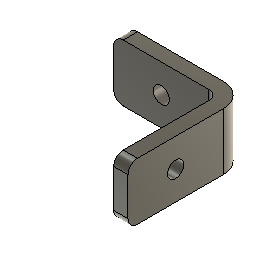
メインロボット ver2 v8 (Autodesk Fusion 360 archive; units mm, degrees)
design "L字固定具"
Autodesk Fusion 360 part; units mm, degrees
sketch "スケッチ1" plane through (0, 0, 0) normal (0, 0, 1) x (1, 0, 0)
  line L0 (0, 0) -> (5, 0)
  line L1 (5, 0) -> (5, 22)
  line L2 (5, 22) -> (0, 22)
  line L3 (0, 22) -> (0, 0)
  line L4 (5, 22) -> (-20, 22)
  line L5 (-20, 22) -> (-20, 25)
  line L6 (-20, 25) -> (5, 25)
  line L7 (5, 25) -> (5, 22)
  constraint horizontal L0
  constraint vertical L1
  constraint horizontal L2
  constraint vertical L3
  constraint coincident L0.start L3.end
  constraint horizontal L4
  constraint vertical L5
  constraint horizontal L6
  constraint vertical L7
extrude "押し出し1" add sketch "スケッチ1" along normal blind 12
sketch "スケッチ2" plane through (5, 0, 0) normal (1, 0, 0) x (0, 1, 0)
  line L0 (0, 0) -> (25, 0)
  line L1 (25, 0) -> (25, 12)
  line L2 (25, 12) -> (0, 12)
  line L3 (0, 12) -> (0, 0)
  line L4 (20, 0) -> (0, 0)
  line L5 (0, 0) -> (0, 12)
  line L6 (0, 12) -> (20, 12)
  line L7 (20, 12) -> (20, 0)
  line L8 (20, 6) -> (0, 6) construction
  line L9 (10, 12) -> (10, 0) construction
  circle A0 centre (10, 6) radius 1.7
  dimension "d3" = 3.4
  constraint horizontal L4
  constraint vertical L5
  constraint horizontal L6
  constraint vertical L7
  constraint coincident L2.end L3.start
  constraint coincident L0 L4.start
  constraint midpoint L7 L8.start
  constraint midpoint L5 L8.end
  constraint midpoint L6 L9.start
  constraint midpoint L4 L9.end
  constraint midpoint L8 A0.centre
  measures "d3" diameter of A0
extrude "押し出し2" cut sketch "スケッチ2" against normal blind 5 contours A0
sketch "スケッチ3" plane through (0, 25, 0) normal (0, 1, 0) x (-1, 0, 0)
  line L0 (-5, 0) -> (20, 0)
  line L1 (20, 0) -> (20, 12)
  line L2 (20, 12) -> (-5, 12)
  line L3 (-5, 12) -> (-5, 0)
  line L4 (0, 0) -> (20, 0)
  line L5 (20, 0) -> (20, 12)
  line L6 (20, 12) -> (0, 12)
  line L7 (0, 12) -> (0, 0)
  line L8 (0, 6) -> (20, 6) construction
  line L9 (10, 12) -> (10, 0) construction
  circle A0 centre (10, 6) radius 1.7
  dimension "d6" = 3.4
  constraint horizontal L4
  constraint vertical L5
  constraint horizontal L6
  constraint vertical L7
  constraint coincident L1.end L2.start
  constraint coincident L4.start L7.end
  constraint midpoint L7 L8.start
  constraint midpoint L5 L8.end
  constraint midpoint L6 L9.start
  constraint midpoint L4 L9.end
  constraint midpoint L9 A0.centre
  measures "d6" diameter of A0
extrude "押し出し3" cut sketch "スケッチ3" against normal blind 5 contours A0
fillet "フィレット1" radius 5 1 edges at (5, 25, 6)
fillet "フィレット1" radius 2 1 edges at (0, 22, 6)
fillet "フィレット1" radius 2 4 edges at (-20, 23.5, 12) (-20, 23.5, 0) (2.5, 0, 12) (2.5, 0, 0)
move_face "面をオフセット1" offset -2 1 faces at (0, 17.2333, 6)

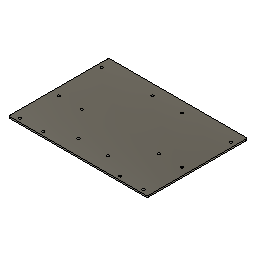
design "下板"
Autodesk Fusion 360 part; units mm, degrees
sketch "スケッチ1" plane through (0, 0, 0) normal (0, 0, 1) x (1, 0, 0)
  line L0 (0, 0) -> (180, 0)
  line L1 (180, 0) -> (180, -100)
  line L2 (180, -100) -> (0, -100)
  line L3 (0, -100) -> (0, 0)
  line L4 (0, -50) -> (180, -50) construction
  line L5 (10, -50) -> (10, -25) construction
  line L6 (10, -25) -> (40, -25) construction
  line L7 (40, -25) -> (40, -50) construction
  line L8 (90, 0) -> (90, -100) construction
  line L9 (10, -50) -> (10, -75) construction
  line L10 (10, -75) -> (40, -75) construction
  line L11 (40, -75) -> (40, -50) construction
  line L12 (140, -75) -> (140, -50) construction
  line L13 (140, -25) -> (140, -50) construction
  line L14 (170, -25) -> (140, -25) construction
  line L15 (170, -50) -> (170, -25) construction
  line L16 (170, -50) -> (170, -75) construction
  line L17 (170, -75) -> (140, -75) construction
  circle A0 centre (10, -25) radius 1.6
  circle A1 centre (40, -25) radius 1.6
  circle A2 centre (10, -75) radius 1.6
  circle A3 centre (40, -75) radius 1.6
  circle A4 centre (170, -25) radius 1.6
  circle A5 centre (140, -25) radius 1.6
  circle A6 centre (140, -75) radius 1.6
  circle A7 centre (170, -75) radius 1.6
  line L18 (40, -37.5) -> (35, -37.5)
  line L19 (35, -37.5) -> (35, -65)
  line L20 (35, -65) -> (45, -65)
  line L21 (45, -65) -> (45, -37.5)
  line L22 (45, -37.5) -> (40, -37.5)
  line L23 (145, -65) -> (135, -65)
  line L24 (135, -65) -> (135, -37.5)
  line L25 (135, -37.5) -> (140, -37.5)
  line L26 (140, -37.5) -> (145, -37.5)
  line L27 (145, -37.5) -> (145, -65)
  line L28 (90, 0) -> (64.5, 0) construction
  line L29 (64.5, 0) -> (64.5, -100) construction
  line L30 (115.5, 0) -> (115.5, -100) construction
  line L31 (64.5, -50) -> (64.5, -9) construction
  line L32 (115.5, -91) -> (115.5, -79)
  circle A8 centre (5, -5) radius 1.6
  circle A9 centre (175, -5) radius 1.6
  circle A10 centre (5, -95) radius 1.6
  circle A11 centre (175, -95) radius 1.6
  line L33 (0, -10) -> (180, -10)
  line L34 (180, -90) -> (0, -90)
  line L35 (0, -80) -> (180, -80)
  line L36 (0, -20) -> (180, -20)
  line L37 (0, 0) -> (180, 0)
  line L38 (180, 0) -> (180, 50)
  line L39 (180, 50) -> (0, 50)
  line L40 (0, 50) -> (0, 0)
  line L41 (90, -60) -> (109.25, -60)
  line L42 (109.25, -60) -> (70.75, -60)
  line L43 (70.75, -60) -> (70.75, 36)
  line L44 (70.75, 36) -> (109.25, 36)
  line L45 (109.25, 36) -> (109.25, -60)
  line L46 (90, -60) -> (90, -80)
  circle A12 centre (70.75, -60) radius 1.6
  circle A13 centre (109.25, -60) radius 1.6
  circle A14 centre (70.75, 36) radius 1.6
  circle A15 centre (109.25, 36) radius 1.6
  line L47 (0, 50) -> (0, 35)
  line L48 (0, 35) -> (180, 35)
  line L49 (0, 35) -> (6, 35)
  circle A16 centre (6, 35) radius 1.6
  circle A17 centre (174, 35) radius 1.6
  dimension "d1" = 180
  dimension "d2" = 100
  dimension "d3" = 3.2
  dimension "d4" = 3.2
  dimension "d7" = 5
  dimension "d8" = 5
  dimension "d9" = 25.5
  dimension "d10" = 41
  dimension "d17" = 3.2
  dimension "d22" = 19.25
  dimension "d23" = 38.5
  dimension "d24" = 96
  dimension "d25" = 20
  dimension "d26" = 3.2
  dimension "d27" = 3.2
  dimension "d28" = 3.2
  dimension "d29" = 3.2
  dimension "d30" = 15
  dimension "d31" = 3.2
  constraint horizontal L0
  constraint vertical L1
  constraint horizontal L2
  constraint vertical L3
  constraint coincident L0.start L3.end
  constraint midpoint L3 L4.start
  constraint midpoint L1 L4.end
  constraint coincident L4 L5.start
  constraint perpendicular L4 L5
  constraint perpendicular L3 L6
  constraint coincident L4 L7.end
  constraint perpendicular L4 L7
  constraint midpoint L0 L8.start
  constraint midpoint L2 L8.end
  constraint symmetric L4 L5.start L9.start
  constraint symmetric L4 L5.end L9.end
  constraint symmetric L4 L6.end L10.end
  constraint symmetric L4 L7.end L11.end
  constraint symmetric L5.start L8 L15.start
  constraint symmetric L5.end L8 L14.start
  constraint symmetric L6.end L8 L13.start
  constraint symmetric L7.end L8 L12.end
  constraint symmetric L8 L5.start L15.start
  constraint symmetric L8 L9.end L16.end
  constraint symmetric L8 L10.end L12.start
  constraint symmetric L8 L7.end L12.end
  constraint coincident L5.end L6.start
  constraint coincident L6.end L7.start
  constraint symmetric L4 A0 A2
  constraint symmetric L4 A1 A3
  constraint symmetric L8 A0 A4
  constraint symmetric L8 A1 A5
  constraint symmetric L8 A2 A7
  constraint symmetric L8 A3 A6
  constraint midpoint L7 L18.start
  constraint perpendicular L7 L18
  constraint perpendicular L4 L19
  constraint perpendicular L11 L20
  constraint perpendicular L20 L21
  constraint perpendicular L7 L22
  constraint symmetric L8 L18.start L25.end
  constraint symmetric L8 L18.end L26.end
  constraint symmetric L8 L19.end L23.start
  constraint symmetric L8 L20.end L23.end
  constraint symmetric L8 L21.end L24.end
  constraint perpendicular L8 L28
  constraint coincident L2 L29.end
  constraint perpendicular L2 L29
  constraint symmetric L8 L28.end L30.start
  constraint symmetric L8 L29.end L30.end
  constraint midpoint L29 L31.start
  constraint perpendicular L4 L31
  constraint symmetric L8 A8 A9
  constraint symmetric L4 A8 A10
  constraint symmetric L4 A9 A11
  constraint coincident L3 L33.start
  constraint coincident L1 L33.end
  constraint perpendicular L1 L33
  constraint coincident L1 L34.start
  constraint coincident L3 L34.end
  constraint perpendicular L3 L34
  constraint coincident L3 L35.start
  constraint coincident L1 L35.end
  constraint perpendicular L1 L35
  constraint coincident L3 L36.start
  constraint coincident L1 L36.end
  constraint perpendicular L1 L36
  constraint horizontal L37
  constraint vertical L38
  constraint horizontal L39
  constraint vertical L40
  constraint coincident L8 L41.start
  constraint perpendicular L30 L41
  constraint horizontal L42
  constraint vertical L43
  constraint horizontal L44
  constraint vertical L45
  constraint midpoint L35 L46.end
  constraint coincident L42.end L43.start
  constraint coincident L41.end L42.start
  constraint coincident L43.end L44.start
  constraint coincident L44.end L45.start
  constraint perpendicular L39 L47
  constraint coincident L38 L48.end
  constraint perpendicular L38 L48
  constraint coincident L48 L49.end
  constraint coincident L49.end A16.centre
  constraint symmetric L8 A16 A17
  measures "d1" distance of L0.start L0.end
  measures "d2" distance of L0.start L2.end
  measures "d3" diameter of A0
  measures "d4" diameter of A1
  measures "d7" distance of L18.start L18.end
  measures "d8" distance of L18.start L21.end
  measures "d9" distance of L8.start L28.end
  measures "d10" distance of L31.start L31.end
  measures "d17" diameter of A8
  measures "d22" distance of L41.start L41.end
  measures "d23" distance of L41.end L42.end
  measures "d24" distance of L41.end L44.end
  measures "d25" distance of L41.start L46.end
  measures "d26" diameter of A12
  measures "d27" diameter of A13
  measures "d28" diameter of A14
  measures "d29" diameter of A15
  measures "d30" distance of L39.end L47.end
  measures "d31" diameter of A16
extrude "押し出し1" add sketch "スケッチ1" along normal blind 2 contours L0 L37 L40 L43 A14 L48 L49 A16 | L0 L3 L33 L37 L43 | L0 L37 L43 L45 A14 A15 L48 | L0 L33 L37 L43 L45 | L3 L33 L36 L43 | L38 L39 L40 L44 A14 A15 L47 L48 L49 A16 A17 | L0 L37 L38 L45 A15 L48 A17 | L0 L1 L33 L37 L45 | L33 L36 L43 L45 | L3 L35 L36 L42 L43 L46 A12 | L1 L33 L36 L45 | L36 L41 L42 L43 L45 A12 A13 | L44 A14 A15 L48 | L1 L35 L36 L41 L42 L45 L46 A13 | L18 L19 L20 L21 L22 | L23 L24 L25 L26 L27 | A8 | A9
fillet "フィレット1" radius 2 4 edges at (0, -80, 1) (180, -80, 1) (0, 50, 1) (180, 50, 1)
equation "d9 = ( 51 / 2 ) * 1 mm"
equation "d10 = ( 82 / 2 ) * 1 mm"
equation "d22 = ( 38.5 / 2 ) * 1 mm"

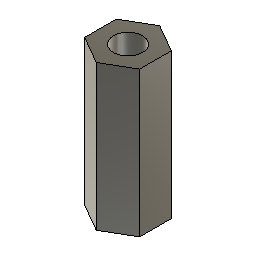
design "15mmスペーサー"
Autodesk Fusion 360 part; units mm, degrees
sketch "スケッチ1" plane through (0, 0, 0) normal (0, 0, 1) x (1, 0, 0)
  line L0 (0, 3.275) -> (-2.8362, 1.6375)
  line L1 (-2.8362, 1.6375) -> (-2.8362, -1.6375)
  line L2 (-2.8362, -1.6375) -> (0, -3.275)
  line L3 (0, -3.275) -> (2.8362, -1.6375)
  line L4 (2.8362, -1.6375) -> (2.8362, 1.6375)
  line L5 (2.8362, 1.6375) -> (0, 3.275)
  circle A0 centre (0, 0) radius 1.5
  dimension "d1" = 3.275
  dimension "d2" = 3
  constraint coincident A0.centre origin
  measures "d1" distance of L0.start A0.centre
  measures "d2" diameter of A0
extrude "押し出し1" add sketch "スケッチ1" along normal blind 15
equation "d1 = ( 6.55 / 2 ) * 1 mm"

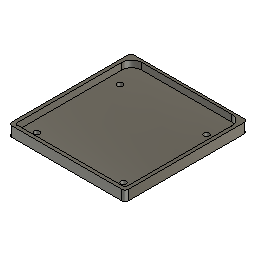
design "基板カバー"
Autodesk Fusion 360 part; units mm, degrees
sketch "スケッチ1" plane through (0, 0, 0) normal (0, 0, 1) x (1, 0, 0)
  line L0 (0, 0) -> (64, 0)
  line L1 (64, 0) -> (64, 70)
  line L2 (64, 70) -> (0, 70)
  line L3 (0, 70) -> (0, 0)
  line L4 (32, 0) -> (32, 5) construction
  line L5 (32, 5) -> (0, 5) construction
  line L6 (0, 5) -> (6, 5)
  circle A0 centre (6, 5) radius 1.6
  line L7 (6, 5) -> (58, 5)
  line L8 (58, 5) -> (58, 55)
  line L9 (58, 55) -> (6, 55)
  line L10 (6, 55) -> (6, 5)
  circle A1 centre (6, 55) radius 1.6
  circle A2 centre (58, 55) radius 1.6
  circle A3 centre (58, 5) radius 1.6
  line L11 (0, 70) -> (-2, 70)
  line L12 (-2, 70) -> (-2, 0)
  line L13 (-2, 0) -> (0, 0)
  line L14 (64, 70) -> (66, 70)
  line L15 (66, 70) -> (66, 0)
  line L16 (66, 0) -> (64, 0)
  line L17 (66, 0) -> (-2, 0)
  line L18 (-2, 0) -> (-2, -2)
  line L19 (-2, -2) -> (66, -2)
  line L20 (66, -2) -> (66, 0)
  line L21 (0, 68) -> (64, 68)
  dimension "d1" = 64
  dimension "d2" = 70
  dimension "d3" = 3.2
  dimension "d4" = 52
  dimension "d5" = 50
  dimension "d6" = 3.2
  dimension "d7" = 3.2
  dimension "d8" = 3.2
  dimension "d16" = 2
  constraint horizontal L0
  constraint vertical L1
  constraint horizontal L2
  constraint vertical L3
  constraint coincident L0.start L3.end
  constraint midpoint L0 L4.start
  constraint perpendicular L0 L4
  constraint coincident L3 L5.end
  constraint perpendicular L3 L5
  constraint coincident L5 L6.end
  constraint coincident L6.end A0.centre
  constraint horizontal L7
  constraint vertical L8
  constraint horizontal L9
  constraint vertical L10
  constraint coincident L9.end L10.start
  constraint coincident L8.end L9.start
  constraint coincident L7.end L8.start
  constraint perpendicular L3 L11
  constraint perpendicular L2 L12
  constraint perpendicular L3 L13
  constraint perpendicular L1 L14
  constraint perpendicular L14 L15
  constraint perpendicular L1 L16
  constraint horizontal L17
  constraint vertical L18
  constraint horizontal L19
  constraint vertical L20
  constraint coincident L3 L21.start
  constraint coincident L1 L21.end
  constraint perpendicular L1 L21
  measures "d1" distance of L0.start L0.end
  measures "d2" distance of L0.start L2.end
  measures "d3" diameter of A0
  measures "d4" distance of L6.end L7.end
  measures "d5" distance of L6.end L9.end
  measures "d6" diameter of A1
  measures "d7" diameter of A2
  measures "d8" diameter of A3
  measures "d16" distance of L1.end L14.end
extrude "押し出し1" add sketch "スケッチ1" along normal blind 2 contours L0 L1 L3 L17 L21 | L3 L11 L12 L13 L17 | L0 L13 L16 L17 L18 L19 L20 | L1 L14 L15 L16 L17 | L1 L2 L3 L21 | A0 L7 L8 L9 L10 A1 A2 A3
extrude "押し出し2" add sketch "スケッチ1" along normal blind 6 contours L3 L11 L12 L13 L17 | L0 L13 L16 L17 L18 L19 L20 | L1 L14 L15 L16 L17 | L1 L2 L3 L21
move_face "面をオフセット2" offset 1 4 faces at (-2, 46, 4) (43.3333, 70, 2) (66, 22, 4) (20.6667, -2, 2)
move_face "面をオフセット3" offset -1 3 faces at (42.6667, 0, 4.6667) (64, 45.3333, 4.6667) (0, 45.3333, 3.3333)
extrude "押し出し3" cut 1 faces at (21, 68, 3.3333) along direction (0, 1, 0) blind 1
fillet "フィレット2" radius 6 2 edges at (-1, 69, 4) (65, 69, 4)
fillet "フィレット2" radius 2 4 edges at (-3, 71, 3) (67, 71, 3) (-3, -3, 3) (67, -3, 3)
fillet "フィレット2" radius 1 2 edges at (65, -1, 4) (-1, -1, 4)
move_face "面をオフセット4" offset -0.5 1 faces at (21, 71, 4)

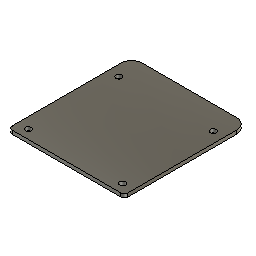
design "基板"
Autodesk Fusion 360 part; units mm, degrees
sketch "スケッチ1" plane through (0, 0, 0) normal (0, 0, 1) x (1, 0, 0)
  line L0 (0, 0) -> (64, 0)
  line L1 (64, 0) -> (64, 70)
  line L2 (64, 70) -> (0, 70)
  line L3 (0, 70) -> (0, 0)
  line L4 (32, 0) -> (32, 5) construction
  line L5 (32, 5) -> (0, 5) construction
  line L6 (0, 5) -> (6, 5)
  circle A0 centre (6, 5) radius 1.6
  line L7 (6, 5) -> (58, 5)
  line L8 (58, 5) -> (58, 55)
  line L9 (58, 55) -> (6, 55)
  line L10 (6, 55) -> (6, 5)
  circle A1 centre (6, 55) radius 1.6
  circle A2 centre (58, 55) radius 1.6
  circle A3 centre (58, 5) radius 1.6
  dimension "d1" = 64
  dimension "d2" = 70
  dimension "d3" = 3.2
  dimension "d4" = 52
  dimension "d5" = 50
  dimension "d6" = 3.2
  dimension "d7" = 3.2
  dimension "d8" = 3.2
  constraint horizontal L0
  constraint vertical L1
  constraint horizontal L2
  constraint vertical L3
  constraint coincident L0.start L3.end
  constraint midpoint L0 L4.start
  constraint perpendicular L0 L4
  constraint coincident L3 L5.end
  constraint perpendicular L3 L5
  constraint coincident L5 L6.end
  constraint coincident L6.end A0.centre
  constraint horizontal L7
  constraint vertical L8
  constraint horizontal L9
  constraint vertical L10
  constraint coincident L9.end L10.start
  constraint coincident L8.end L9.start
  constraint coincident L7.end L8.start
  measures "d1" distance of L0.start L0.end
  measures "d2" distance of L0.start L2.end
  measures "d3" diameter of A0
  measures "d4" distance of L6.end L7.end
  measures "d5" distance of L6.end L9.end
  measures "d6" diameter of A1
  measures "d7" diameter of A2
  measures "d8" diameter of A3
extrude "押し出し1" add sketch "スケッチ1" along normal blind 2 contours L0 L1 L2 L3 | A0 L7 L8 L9 L10 A1 A2 A3
fillet "フィレット1" radius 2 2 edges at (0, 0, 1) (64, 0, 1)
fillet "フィレット1" radius 6 2 edges at (0, 70, 1) (64, 70, 1)
move_face "面をオフセット1" offset -2 1 faces at (40.6667, 70, 0.6667)
sketch "スケッチ2" plane through (0, 0, 2) normal (0, 0, 1) x (-1, 0, 0)
  arc A0 (-6, -68) -> (0, -62) centre (-6, -62) ccw
  line L0 (0, -62) -> (0, -2)
  arc A1 (0, -2) -> (-2, 0) centre (-2, -2) ccw
  line L1 (-2, 0) -> (-62, 0)
  arc A2 (-62, 0) -> (-64, -2) centre (-62, -2) ccw
  line L2 (-64, -2) -> (-64, -62)
  arc A3 (-64, -62) -> (-58, -68) centre (-58, -62) ccw
  line L3 (-58, -68) -> (-6, -68)
  circle A4 centre (-58, -5) radius 1.6
  circle A5 centre (-6, -55) radius 1.6
  circle A6 centre (-6, -5) radius 1.6
  circle A7 centre (-58, -55) radius 1.6

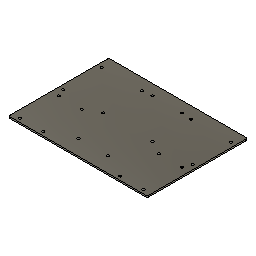
design "上板"
Autodesk Fusion 360 part; units mm, degrees
sketch "スケッチ1" plane through (0, 0, 0) normal (0, 0, 1) x (1, 0, 0)
  line L0 (0, 0) -> (180, 0)
  line L1 (180, 0) -> (180, -100)
  line L2 (180, -100) -> (0, -100)
  line L3 (0, -100) -> (0, 0)
  line L4 (0, -50) -> (180, -50) construction
  line L5 (10, -50) -> (10, -25) construction
  line L6 (10, -25) -> (40, -25) construction
  line L7 (40, -25) -> (40, -50) construction
  line L8 (90, 0) -> (90, -100) construction
  line L9 (10, -50) -> (10, -75) construction
  line L10 (10, -75) -> (40, -75) construction
  line L11 (40, -75) -> (40, -50) construction
  line L12 (140, -75) -> (140, -50) construction
  line L13 (140, -25) -> (140, -50) construction
  line L14 (170, -25) -> (140, -25) construction
  line L15 (170, -50) -> (170, -25) construction
  line L16 (170, -50) -> (170, -75) construction
  line L17 (170, -75) -> (140, -75) construction
  circle A0 centre (10, -25) radius 1.6
  circle A1 centre (40, -25) radius 1.6
  circle A2 centre (10, -75) radius 1.6
  circle A3 centre (40, -75) radius 1.6
  circle A4 centre (170, -25) radius 1.6
  circle A5 centre (140, -25) radius 1.6
  circle A6 centre (140, -75) radius 1.6
  circle A7 centre (170, -75) radius 1.6
  line L18 (40, -37.5) -> (35, -37.5)
  line L19 (35, -37.5) -> (35, -65)
  line L20 (35, -65) -> (45, -65)
  line L21 (45, -65) -> (45, -37.5)
  line L22 (45, -37.5) -> (40, -37.5)
  line L23 (145, -65) -> (135, -65)
  line L24 (135, -65) -> (135, -37.5)
  line L25 (135, -37.5) -> (140, -37.5)
  line L26 (140, -37.5) -> (145, -37.5)
  line L27 (145, -37.5) -> (145, -65)
  line L28 (90, 0) -> (64.5, 0) construction
  line L29 (64.5, 0) -> (64.5, -100) construction
  line L30 (115.5, 0) -> (115.5, -100) construction
  line L31 (64.5, -50) -> (64.5, -9) construction
  line L32 (115.5, -91) -> (115.5, -79)
  circle A8 centre (5, -95) radius 1.6
  circle A9 centre (175, -95) radius 1.6
  line L33 (0, -10) -> (180, -10)
  line L34 (180, -90) -> (0, -90)
  line L35 (0, -80) -> (180, -80)
  line L36 (0, -20) -> (180, -20)
  line L37 (0, 0) -> (180, 0)
  line L38 (180, 0) -> (180, 50)
  line L39 (180, 50) -> (0, 50)
  line L40 (0, 50) -> (0, 0)
  line L41 (90, -80) -> (90, -60)
  line L42 (90, -60) -> (109.25, -60)
  line L43 (109.25, -60) -> (70.75, -60)
  line L44 (70.75, -60) -> (70.75, 36)
  line L45 (70.75, 36) -> (109.25, 36)
  line L46 (109.25, 36) -> (109.25, -60)
  circle A10 centre (70.75, 36) radius 1.6
  circle A11 centre (109.25, 36) radius 1.6
  circle A12 centre (70.75, -60) radius 1.6
  circle A13 centre (109.25, -60) radius 1.6
  line L47 (180, 50) -> (180, 35)
  line L48 (180, 35) -> (0, 35)
  line L49 (0, 35) -> (6, 35)
  circle A14 centre (6, 35) radius 1.6
  circle A15 centre (174, 35) radius 1.6
  line L50 (6, 35) -> (58, 35)
  line L51 (58, 35) -> (58, -15)
  line L52 (58, -15) -> (6, -15)
  line L53 (6, -15) -> (6, 35)
  circle A16 centre (6, -15) radius 1.6
  circle A17 centre (58, -15) radius 1.6
  circle A18 centre (58, 35) radius 1.6
  circle A19 centre (122, 35) radius 1.6
  circle A20 centre (174, 35) radius 1.6
  circle A21 centre (174, -15) radius 1.6
  circle A22 centre (122, -15) radius 1.6
  line L54 (122, 35) -> (122, -15)
  line L55 (174, -15) -> (174, 35)
  line L56 (174, 35) -> (122, 35)
  line L57 (122, -15) -> (174, -15)
  line L58 (58, 35) -> (64, 35)
  line L59 (64, 35) -> (64, 50)
  line L60 (64, 50) -> (0, 50)
  line L61 (0, 50) -> (0, -20)
  line L62 (0, -20) -> (64, -20)
  line L63 (64, -20) -> (64, 50)
  dimension "d1" = 180
  dimension "d2" = 100
  dimension "d3" = 3.2
  dimension "d4" = 3.2
  dimension "d7" = 5
  dimension "d8" = 5
  dimension "d9" = 25.5
  dimension "d10" = 41
  dimension "d22" = 20
  dimension "d23" = 19.25
  dimension "d24" = 38.5
  dimension "d25" = 96
  dimension "d26" = 3.2
  dimension "d27" = 3.2
  dimension "d28" = 3.2
  dimension "d29" = 3.2
  dimension "d30" = 15
  dimension "d31" = 6
  dimension "d32" = 3.2
  dimension "d33" = 52
  dimension "d34" = 50
  dimension "d35" = 3.2
  dimension "d36" = 3.2
  dimension "d37" = 3.2
  dimension "d38" = 70
  constraint horizontal L0
  constraint vertical L1
  constraint horizontal L2
  constraint vertical L3
  constraint coincident L0.start L3.end
  constraint midpoint L3 L4.start
  constraint midpoint L1 L4.end
  constraint coincident L4 L5.start
  constraint perpendicular L4 L5
  constraint perpendicular L3 L6
  constraint coincident L4 L7.end
  constraint perpendicular L4 L7
  constraint midpoint L0 L8.start
  constraint midpoint L2 L8.end
  constraint symmetric L4 L5.start L9.start
  constraint symmetric L4 L5.end L9.end
  constraint symmetric L4 L6.end L10.end
  constraint symmetric L4 L7.end L11.end
  constraint symmetric L5.start L8 L15.start
  constraint symmetric L5.end L8 L14.start
  constraint symmetric L6.end L8 L13.start
  constraint symmetric L7.end L8 L12.end
  constraint symmetric L8 L5.start L15.start
  constraint symmetric L8 L9.end L16.end
  constraint symmetric L8 L10.end L12.start
  constraint symmetric L8 L7.end L12.end
  constraint coincident L5.end L6.start
  constraint coincident L6.end L7.start
  constraint symmetric L4 A0 A2
  constraint symmetric L4 A1 A3
  constraint symmetric L8 A0 A4
  constraint symmetric L8 A1 A5
  constraint symmetric L8 A2 A7
  constraint symmetric L8 A3 A6
  constraint midpoint L7 L18.start
  constraint perpendicular L7 L18
  constraint perpendicular L4 L19
  constraint perpendicular L11 L20
  constraint perpendicular L20 L21
  constraint perpendicular L7 L22
  constraint symmetric L8 L18.start L25.end
  constraint symmetric L8 L18.end L26.end
  constraint symmetric L8 L19.end L23.start
  constraint symmetric L8 L20.end L23.end
  constraint symmetric L8 L21.end L24.end
  constraint perpendicular L8 L28
  constraint coincident L2 L29.end
  constraint perpendicular L2 L29
  constraint symmetric L8 L28.end L30.start
  constraint symmetric L8 L29.end L30.end
  constraint midpoint L29 L31.start
  constraint perpendicular L4 L31
  constraint coincident L3 L33.start
  constraint coincident L1 L33.end
  constraint perpendicular L1 L33
  constraint coincident L1 L34.start
  constraint coincident L3 L34.end
  constraint perpendicular L3 L34
  constraint coincident L3 L35.start
  constraint coincident L1 L35.end
  constraint perpendicular L1 L35
  constraint coincident L3 L36.start
  constraint coincident L1 L36.end
  constraint perpendicular L1 L36
  constraint horizontal L37
  constraint vertical L38
  constraint horizontal L39
  constraint vertical L40
  constraint midpoint L35 L41.start
  constraint perpendicular L35 L41
  constraint perpendicular L41 L42
  constraint horizontal L43
  constraint vertical L44
  constraint horizontal L45
  constraint vertical L46
  constraint coincident L44.end L45.start
  constraint coincident L45.end L46.start
  constraint coincident L43.end L44.start
  constraint coincident L42.end L43.start
  constraint perpendicular L39 L47
  constraint coincident L40 L48.end
  constraint perpendicular L40 L48
  constraint perpendicular L40 L49
  constraint coincident L49.end A14.centre
  constraint symmetric L8 A14 A15
  constraint horizontal L50
  constraint vertical L51
  constraint horizontal L52
  constraint vertical L53
  constraint coincident L52.end L53.start
  constraint coincident L51.end L52.start
  constraint coincident L50.end L51.start
  constraint symmetric L8 A14 A20
  constraint symmetric L8 L49.end A15.centre
  constraint symmetric L8 L50.end A19.centre
  constraint symmetric L8 L51.end A22.centre
  constraint symmetric L8 L52.end A21.centre
  constraint symmetric L8 A16 A21
  constraint symmetric L8 A17 A22
  constraint symmetric L8 A18 A19
  constraint coincident L48 L58.end
  constraint coincident L39 L59.end
  constraint perpendicular L39 L59
  constraint horizontal L60
  constraint vertical L61
  constraint horizontal L62
  constraint vertical L63
  measures "d1" distance of L0.start L0.end
  measures "d2" distance of L0.start L2.end
  measures "d3" diameter of A0
  measures "d4" diameter of A1
  measures "d7" distance of L18.start L18.end
  measures "d8" distance of L18.start L21.end
  measures "d9" distance of L8.start L28.end
  measures "d10" distance of L31.start L31.end
  measures "d22" distance of L41.start L41.end
  measures "d23" distance of L41.end L42.end
  measures "d24" distance of L42.end L43.end
  measures "d25" distance of L42.end L45.end
  measures "d26" diameter of A10
  measures "d27" diameter of A11
  measures "d28" diameter of A12
  measures "d29" diameter of A13
  measures "d30" distance of L38.end L47.end
  measures "d31" distance of L48.end L49.end
  measures "d32" diameter of A14
  measures "d33" distance of L49.end L50.end
  measures "d34" distance of L49.end L52.end
  measures "d35" diameter of A16
  measures "d36" diameter of A17
  measures "d37" diameter of A18
  measures "d38" distance of L59.end L62.end
extrude "押し出し1" add sketch "スケッチ1" along normal blind 2 contours L0 L37 L40 L48 L49 A14 L53 L61 | L0 L3 L33 L37 L53 L61 | L0 L37 L48 A14 L50 L51 L53 A18 | L0 L33 L37 L51 L53 | L3 L33 L36 L51 L52 L53 A16 A17 L61 L62 L63 | L39 L40 L48 L49 A14 L50 A18 L58 L59 L60 L61 L63 | L0 L37 L48 L51 A18 L58 L63 | L0 L33 L37 L51 L63 | L33 L51 L52 L53 A16 A17 | L3 L35 L36 L41 L43 L44 A12 L62 | L0 L37 L44 A10 L48 L63 | L0 L33 L37 L44 L63 | L33 L36 L44 L63 | L38 L39 L45 A10 A11 L47 L48 A15 A19 A20 L56 L59 L63 | L0 L37 L44 L46 A10 A11 L48 | L0 L33 L37 L44 L46 | L1 L35 L36 L41 L42 L43 L46 A13 | L33 L36 L44 L46 | L36 L42 L43 L44 L46 A12 A13 | L0 L37 L46 A11 L48 A19 L54 | L0 L33 L37 L46 L54 | L1 L33 L36 L46 A21 A22 L54 L55 L57 | L0 L37 L38 L48 A15 A20 L55 | L0 L37 L48 A15 A19 A20 L54 L55 L56 | L0 L33 L37 L54 L55 | L45 A10 A11 L48 | L0 L1 L33 L37 L55 | L33 A21 A22 L54 L55 L57 | L18 L19 L20 L21 L22 | L23 L24 L25 L26 L27
fillet "フィレット1" radius 2 4 edges at (0, -80, 1) (180, -80, 1) (0, 50, 1) (180, 50, 1)
equation "d9 = ( 51 / 2 ) * 1 mm"
equation "d10 = ( 82 / 2 ) * 1 mm"

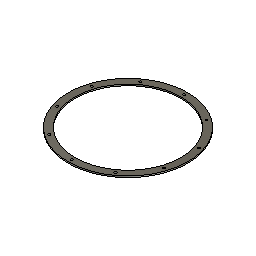
design "バスケットリング"
Autodesk Fusion 360 part; units mm, degrees
sketch "スケッチ1" plane through (0, 0, 0) normal (0, 0, 1) x (1, 0, 0)
  circle A0 centre (0, 0) radius 75
  circle A1 centre (0, 0) radius 85
  line L0 (0, 75) -> (0, 85)
  circle A2 centre (0, 80) radius 1.6
  circle A3 centre (-47.0228, 64.7214) radius 1.6
  circle A4 centre (-76.0845, 24.7214) radius 1.6
  circle A5 centre (-76.0845, -24.7214) radius 1.6
  circle A6 centre (-47.0228, -64.7214) radius 1.6
  circle A7 centre (0, -80) radius 1.6
  circle A8 centre (47.0228, -64.7214) radius 1.6
  circle A9 centre (76.0845, -24.7214) radius 1.6
  circle A10 centre (76.0845, 24.7214) radius 1.6
  circle A11 centre (47.0228, 64.7214) radius 1.6
  dimension "d1" = 150
  dimension "d4" = 170
  dimension "d7" = 3.2
  dimension "d9" = 360
  constraint coincident A0.centre A1.centre
  constraint concentric A0 A1
  constraint coincident A0 L0.start
  constraint coincident A1 L0.end
  constraint vertical L0
  constraint midpoint L0 A2.centre
  measures "d1" diameter of A0
  measures "d4" diameter of A1
  measures "d7" diameter of A2
extrude "押し出し1" add sketch "スケッチ1" along normal blind 2
extrude "押し出し2" [rolled back] along distance -10 taper angle 0

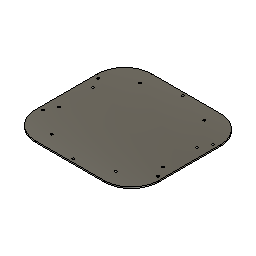
design "バスケット底"
Autodesk Fusion 360 part; units mm, degrees
sketch "スケッチ1" plane through (0, 0, 0) normal (0, 0, 1) x (1, 0, 0)
  circle A0 centre (0, 0) radius 75
  circle A1 centre (0, 0) radius 85
  line L0 (0, 75) -> (0, 85)
  circle A2 centre (0, 80) radius 1.6
  circle A3 centre (-47.0228, 64.7214) radius 1.6
  circle A4 centre (-76.0845, 24.7214) radius 1.6
  circle A5 centre (-76.0845, -24.7214) radius 1.6
  circle A6 centre (-47.0228, -64.7214) radius 1.6
  circle A7 centre (0, -80) radius 1.6
  circle A8 centre (47.0228, -64.7214) radius 1.6
  circle A9 centre (76.0845, -24.7214) radius 1.6
  circle A10 centre (76.0845, 24.7214) radius 1.6
  circle A11 centre (47.0228, 64.7214) radius 1.6
  line L1 (0, 0) -> (-84, 0)
  line L2 (-84, 0) -> (-84, -40.186)
  line L3 (0, 0) -> (0, 85)
  line L4 (84, 0) -> (84, -40.186)
  line L5 (-84, 0) -> (-84, 40.186)
  line L6 (84, 0) -> (84, 40.186)
  circle A12 centre (-84, 40.186) radius 1.6
  circle A13 centre (84, 40.186) radius 1.6
  circle A14 centre (-84, -40.186) radius 1.6
  circle A15 centre (84, -40.186) radius 1.6
  line L7 (0, 85) -> (-90, 85)
  line L8 (-90, 85) -> (-90, 0)
  line L9 (-90, 0) -> (0, 0)
  line L10 (0, 0) -> (0, 85)
  line L11 (90, 85) -> (90, 0)
  line L12 (0, 85) -> (90, 85)
  line L13 (-90, -85) -> (-90, 0)
  line L14 (0, -85) -> (-90, -85)
  line L15 (0, -85) -> (90, -85)
  line L16 (90, -85) -> (90, 0)
  dimension "d1" = 150
  dimension "d4" = 170
  dimension "d7" = 3.2
  dimension "d9" = 360
  dimension "d10" = 84
  dimension "d11" = 40.186
  dimension "d12" = 3.2
  dimension "d13" = 3.2
  dimension "d14" = 3.2
  dimension "d15" = 3.2
  constraint coincident A0.centre A1.centre
  constraint concentric A0 A1
  constraint coincident A0 L0.start
  constraint coincident A1 L0.end
  constraint vertical L0
  constraint midpoint L0 A2.centre
  constraint horizontal L1
  constraint perpendicular L1 L2
  constraint parallel L0 L3
  constraint symmetric L1.end L3 L4.start
  constraint symmetric L2.end L3 L4.end
  constraint symmetric L2.start L1 L5.start
  constraint symmetric L1 L2.end L5.end
  constraint symmetric L1 L4.start L6.start
  constraint symmetric L1 L4.end L6.end
  constraint coincident L5.end A12.centre
  constraint coincident L6.end A13.centre
  constraint coincident L2.end A14.centre
  constraint coincident L4.end A15.centre
  constraint horizontal L7
  constraint vertical L8
  constraint horizontal L9
  constraint vertical L10
  constraint symmetric L0.end L3 L7.start
  constraint symmetric L3 L7.end L11.start
  constraint symmetric L3 L8.end L11.end
  constraint symmetric L0.end L9 L14.start
  constraint symmetric L7.end L9 L13.start
  constraint symmetric L8.end L9 L13.end
  constraint symmetric L9 L11.start L15.end
  constraint symmetric L9 L11.end L16.end
  constraint symmetric L9 L0.end L14.start
  measures "d1" diameter of A0
  measures "d4" diameter of A1
  measures "d7" diameter of A2
  measures "d10" distance of A0.centre L1.end
  measures "d11" distance of L1.end L2.end
  measures "d12" diameter of A12
  measures "d13" diameter of A13
  measures "d14" diameter of A14
  measures "d15" diameter of A15
extrude "押し出し1" add sketch "スケッチ1" along normal blind 2 contours A0 L1 L3 L9 L10 | A0 A1 L0 A2 L1 L2 L3 L4 L6 L9 L10 | A0 L1 L3 L9 L10 | A0 A1 L0 A2 L1 L3 L5 L9 L10 | A1 L5 L9 | A1 L2 L9 | A1 L9 L13 L14 | A1 L7 L8 L9 | A1 L11 L12 L15 L16 | A1 L4 L6
fillet "フィレット1" radius 40 4 edges at (-90, -85, 1) (90, -85, 1) (90, 85, 1) (-90, 85, 1)
equation "d10 = ( 168 / 2 ) * 1 mm"
equation "d11 = ( 80.372 / 2 ) * 1 mm"

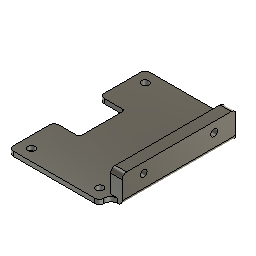
design "モーター固定具"
Autodesk Fusion 360 part; units mm, degrees
sketch "スケッチ1" plane through (0, 0, 0) normal (0, 0, 1) x (1, 0, 0)
  line L0 (19.8573, -35) -> (-20, -35)
  line L1 (-20, -35) -> (-20, 35)
  line L2 (-20, 35) -> (19.8573, 35)
  line L3 (19.8573, 35) -> (19.8573, -35)
  line L4 (0, -25) -> (-20, -25)
  line L5 (0, -25) -> (19.8573, -25)
  circle A0 centre (-15, -25) radius 1.6
  circle A1 centre (15, -25) radius 1.6
  line L6 (1.75, 0) -> (22.5, 0)
  circle A2 centre (15, 25) radius 1.6
  line L7 (0, 25) -> (19.8573, 25)
  circle A3 centre (-15, 25) radius 1.6
  line L8 (0, 25) -> (-20, 25)
  line L9 (-13, -10) -> (-20, -10)
  line L10 (-20, -10) -> (-20, 10)
  line L11 (-20, 10) -> (-13, 10)
  line L12 (-13, -10) -> (-9, -10)
  line L13 (-9, -10) -> (-9, 10)
  line L14 (-9, 10) -> (-13, 10)
  line L15 (-0.1427, -30) -> (-20, -30)
  line L16 (-0.1427, -30) -> (19.8573, -30)
  line L17 (-0.1427, 30) -> (-20, 30)
  line L18 (-0.1427, 30) -> (19.8573, 30)
  point P0 (-15, 25)
  dimension "d1" = 3.2
  dimension "d2" = 3.2
  dimension "d7" = 7
  dimension "d8" = 20
  dimension "d13" = 4
  constraint horizontal L0
  constraint vertical L1
  constraint horizontal L2
  constraint vertical L3
  constraint coincident L1 L4.end
  constraint perpendicular L1 L4
  constraint coincident L3 L5.end
  constraint perpendicular L3 L5
  constraint symmetric L4.start L6 L7.start
  constraint symmetric L5.end L6 L7.end
  constraint symmetric A0.centre L6 P0
  constraint symmetric A1 L6 A2
  constraint symmetric L4.end L6 L8.end
  constraint symmetric A0 L6 A3
  constraint horizontal L9
  constraint vertical L10
  constraint horizontal L11
  constraint horizontal L12
  constraint vertical L13
  constraint horizontal L14
  constraint coincident L4 A0.centre
  constraint coincident L5 A1.centre
  constraint coincident L1 L15.end
  constraint perpendicular L1 L15
  constraint coincident L3 L16.end
  constraint perpendicular L3 L16
  constraint coincident L1 L17.end
  constraint perpendicular L1 L17
  constraint coincident L3 L18.end
  constraint perpendicular L3 L18
  measures "d1" diameter of A0
  measures "d2" diameter of A1
  measures "d7" distance of L9.start L9.end
  measures "d8" distance of L9.start L11.end
  measures "d13" distance of L9.start L12.end
extrude "押し出し1" add sketch "スケッチ1" against normal blind 2 contours L1 L3 L4 L5 A0 A1 L15 L16 | L1 L3 L4 L5 A0 A1 A2 L7 A3 L8 L9 L11 L12 L13 L14 | L1 L3 A2 L7 A3 L8 L17 L18
sketch "スケッチ2" plane through (19.8573, 0, 0) normal (1, 0, 0) x (0, 1, 0)
  line L0 (15.4432, 42.3359) -> (-15.5568, 42.3359)
  line L1 (-15.5568, 42.3359) -> (-21.2068, 36.6859)
  line L2 (-21.2068, 36.6859) -> (-21.2068, 5.6859)
  line L3 (-21.2068, 5.6859) -> (-15.5568, 0.0359)
  line L4 (-15.5568, 0.0359) -> (15.4432, 0.0359)
  line L5 (15.4432, 0.0359) -> (21.0932, 5.6859)
  line L6 (21.0932, 5.6859) -> (21.0932, 36.6859)
  line L7 (21.0932, 36.6859) -> (15.4432, 42.3359)
  circle A0 centre (-15.5568, 36.6859) radius 1.5
  circle A1 centre (-15.5568, 5.6859) radius 1.5
  circle A2 centre (15.4432, 5.6859) radius 1.5
  circle A3 centre (15.4432, 36.6859) radius 1.5
  circle A4 centre (-0.0568, 21.1859) radius 11
  circle A5 centre (-15.5568, 5.6859) radius 1.5
  circle A6 centre (15.4432, 5.6859) radius 1.5
  line L8 (-25, 10) -> (25, 10)
  line L9 (25, 10) -> (25, 0)
  line L10 (25, 0) -> (-25, 0)
  line L11 (-25, 0) -> (-25, 10)
  line L12 (-25, 0) -> (25, 0)
  line L13 (25, 0) -> (25, -2)
  line L14 (25, -2) -> (-25, -2)
  line L15 (-25, -2) -> (-25, 0)
  constraint concentric A1 A5
  constraint concentric A2 A6
  constraint horizontal L8
  constraint vertical L9
  constraint horizontal L10
  constraint vertical L11
  constraint horizontal L12
  constraint vertical L13
  constraint horizontal L14
  constraint vertical L15
extrude "押し出し2" add sketch "スケッチ2" along normal blind 5 contours L2 L3 L4 L5 L6 L8 L9 L10 L11 L12 | L2 L3 L4 L5 L6 L8 | L10 L12 L13 L14 L15
fillet "フィレット1" radius 3 2 edges at (19.8573, 25, -1) (19.8573, -25, -1)
fillet "フィレット1" radius 2 8 edges at (22.3573, -25, 10) (22.3573, 25, 10) (-20, 10, -1) (-20, -10, -1) (-20, -30, -1) (19.8573, -30, -1) (-20, 30, -1) (19.8573, 30, -1)
fillet "フィレット1" radius 1 2 edges at (-9, 10, -1) (-9, -10, -1)
fillet "フィレット2" radius 2 1 edges at (24.8573, 0, -2)

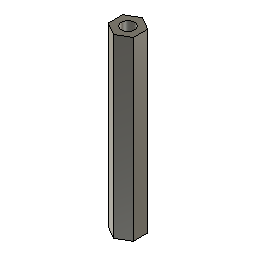
design "40mmスペーサー"
Autodesk Fusion 360 part; units mm, degrees
sketch "スケッチ1" plane through (0, 0, 0) normal (0, 0, 1) x (1, 0, 0)
  line L0 (0, 3.275) -> (-2.8362, 1.6375)
  line L1 (-2.8362, 1.6375) -> (-2.8362, -1.6375)
  line L2 (-2.8362, -1.6375) -> (0, -3.275)
  line L3 (0, -3.275) -> (2.8362, -1.6375)
  line L4 (2.8362, -1.6375) -> (2.8362, 1.6375)
  line L5 (2.8362, 1.6375) -> (0, 3.275)
  circle A0 centre (0, 0) radius 1.5
  dimension "d1" = 3.275
  dimension "d2" = 3
  constraint coincident A0.centre origin
  measures "d1" distance of L0.start A0.centre
  measures "d2" diameter of A0
extrude "押し出し1" add sketch "スケッチ1" along normal blind 40
equation "d1 = ( 6.55 / 2 ) * 1 mm"
